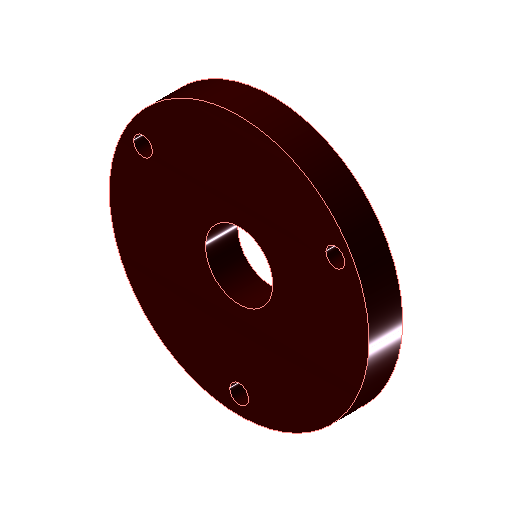
# Autodesk Inventor part: 50_ETL_Lid_v0
Saved by Autodesk Inventor 2022 (Build 260153000, 153)
## iProperties
Created: 2021-12-31
Part Number: 50_ETL_Lid_v0
Material: Generisch
Document SubType Name: Modeling
Designer: diederichbenedict
Density: 1 g/cm^3
Appearance: Orangerot
Author: diederichbenedict
Autodesk Inventor part; units mm, degrees
ref_plane "YZ Plane" through (0, 0, 0) normal (1, 0, 0) x (0, 1, 0)
ref_plane "XZ Plane" through (0, 0, 0) normal (0, 1, 0) x (-1, 0, 0)
ref_plane "XY Plane" through (0, 0, 0) normal (0, 0, 1) x (1, 0, 0)
sketch "Skizze1" plane through (0, 0, 0) normal (0, 1, 0) x (-1, 0, 0)
  line L0 (-3.6106, 0) -> (-3.6106, -12.505)
  line L1 (-38.6, 0) -> (0, 0) projected
  line L2 (-13.05, -7.505) -> (-13.05, -21.905) projected
  line L3 (-25.55, -7.505) -> (-25.55, -21.905) projected
  line L4 (-6.3, -0.4913) -> (-6.3, 0)
  line L5 (-32.3, -0.4913) -> (-6.3, -0.4913) projected
  line L6 (0, 0) -> (0, 5)
  line L7 (0, 5) -> (-14.3, 5)
  line L8 (-14.3, 5) -> (-14.3, 0.2)
  line L9 (-14.3, 0.2) -> (-6.65, 0.2)
  line L10 (-6.65, 0.2) -> (-6.65, 0)
  line L11 (0, 0) -> (-6.65, 0)
  line L12 (-19.3, -19.905) -> (-19.3, 13.9284)
  dimension "d0" = 5
  dimension "d1" = 12.65
  dimension "d2" = 12.5
  dimension "d3" = 6.25
  dimension "d4" = 0.2
  dimension "d6" = 5
  constraints: 18 end point, 4 perpendicular, 4 vertical, 1 point on line, 4 other
  measures "d0" distance of L1.end L6.end
  measures "d1" distance from line of L12 L9.end
  measures "d2" distance between parallel lines of L3 L2
  measures "d3" distance between parallel lines of L12 L2
  measures "d4" distance between parallel lines of L9 L1
  measures "d6" distance between parallel lines of L8 L12
revolve "Umdrehung1" add sketch "Skizze1" angle 360 about axis through (19.3, 0, -19.905) along (0, 0, 1) contours L10 L9 L8 L7 L6 L1
sketch "Skizze2" plane through (19.3, 0, 5) normal (0, 0, 1) x (1, 0, 0)
  circle A0 centre (0, -16.5) radius 1.4 projected
  circle A1 centre (0, 0) radius 19.3 projected
  circle A2 centre (0, 0) radius 12.65 projected
  circle A3 centre (-14.2894, 8.25) radius 1.4 projected
  circle A4 centre (14.2894, 8.25) radius 1.4 projected
  point P0 (-19.3, 0)
extrude "Extrusion1" cut sketch "Skizze2" against normal through all contours A0 | A3 | A4
equation "\"d3\" = 0.5 * d2"
